Autodesk Inventor part; units mm, degrees
(part 3 of 6)
  line L1824 (13.0001, 24.773) -> (14.0001, 24.773)
  line L1825 (14.0001, 24.773) -> (14.0001, 25.773)
  line L1826 (14.0001, 25.773) -> (13.0001, 25.773)
  line L1827 (13.0001, 25.773) -> (13.0001, 24.773)
  line L1828 (13.8383, 24.773) -> (14.8383, 24.773)
  line L1829 (14.8383, 24.773) -> (14.8383, 25.773)
  line L1830 (14.8383, 25.773) -> (13.8383, 25.773)
  line L1831 (13.8383, 25.773) -> (13.8383, 24.773)
  line L1832 (14.6765, 24.773) -> (15.6765, 24.773)
  line L1833 (15.6765, 24.773) -> (15.6765, 25.773)
  line L1834 (15.6765, 25.773) -> (14.6765, 25.773)
  line L1835 (14.6765, 25.773) -> (14.6765, 24.773)
  line L1836 (15.4766, 24.773) -> (16.4766, 24.773)
  line L1837 (16.4766, 24.773) -> (16.4766, 25.773)
  line L1838 (16.4766, 25.773) -> (15.4766, 25.773)
  line L1839 (15.4766, 25.773) -> (15.4766, 24.773)
  line L1840 (15.9973, 24.773) -> (16.9973, 24.773)
  line L1841 (16.9973, 24.773) -> (16.9973, 25.773)
  line L1842 (16.9973, 25.773) -> (15.9973, 25.773)
  line L1843 (15.9973, 25.773) -> (15.9973, 24.773)
  line L1844 (17.153, 24.773) -> (18.153, 24.773)
  line L1845 (18.153, 24.773) -> (18.153, 25.773)
  line L1846 (18.153, 25.773) -> (17.153, 25.773)
  line L1847 (17.153, 25.773) -> (17.153, 24.773)
  line L1848 (17.915, 24.773) -> (18.915, 24.773)
  line L1849 (18.915, 24.773) -> (18.915, 25.773)
  line L1850 (18.915, 25.773) -> (17.915, 25.773)
  line L1851 (17.915, 25.773) -> (17.915, 24.773)
  line L1852 (18.677, 24.773) -> (19.677, 24.773)
  line L1853 (19.677, 24.773) -> (19.677, 25.773)
  line L1854 (19.677, 25.773) -> (18.677, 25.773)
  line L1855 (18.677, 25.773) -> (18.677, 24.773)
  line L1856 (19.2358, 24.773) -> (20.2358, 24.773)
  line L1857 (20.2358, 24.773) -> (20.2358, 25.773)
  line L1858 (20.2358, 25.773) -> (19.2358, 25.773)
  line L1859 (19.2358, 25.773) -> (19.2358, 24.773)
  line L1860 (19.8327, 24.773) -> (20.8327, 24.773)
  line L1861 (20.8327, 24.773) -> (20.8327, 25.773)
  line L1862 (20.8327, 25.773) -> (19.8327, 25.773)
  line L1863 (19.8327, 25.773) -> (19.8327, 24.773)
  line L1864 (20.4677, 24.773) -> (21.4677, 24.773)
  line L1865 (21.4677, 24.773) -> (21.4677, 25.773)
  line L1866 (21.4677, 25.773) -> (20.4677, 25.773)
  line L1867 (20.4677, 25.773) -> (20.4677, 24.773)
  line L1868 (21.471, 24.773) -> (22.471, 24.773)
  line L1869 (22.471, 24.773) -> (22.471, 25.773)
  line L1870 (22.471, 25.773) -> (21.471, 25.773)
  line L1871 (21.471, 25.773) -> (21.471, 24.773)
  line L1872 (12.9874, 24.7984) -> (13.9874, 24.7984)
  line L1873 (13.9874, 24.7984) -> (13.9874, 25.7984)
  line L1874 (13.9874, 25.7984) -> (12.9874, 25.7984)
  line L1875 (12.9874, 25.7984) -> (12.9874, 24.7984)
  line L1876 (13.8256, 24.7984) -> (14.8256, 24.7984)
  line L1877 (14.8256, 24.7984) -> (14.8256, 25.7984)
  line L1878 (14.8256, 25.7984) -> (13.8256, 25.7984)
  line L1879 (13.8256, 25.7984) -> (13.8256, 24.7984)
  line L1880 (14.6765, 24.7984) -> (15.6765, 24.7984)
  line L1881 (15.6765, 24.7984) -> (15.6765, 25.7984)
  line L1882 (15.6765, 25.7984) -> (14.6765, 25.7984)
  line L1883 (14.6765, 25.7984) -> (14.6765, 24.7984)
  line L1884 (15.4766, 24.7984) -> (16.4766, 24.7984)
  line L1885 (16.4766, 24.7984) -> (16.4766, 25.7984)
  line L1886 (16.4766, 25.7984) -> (15.4766, 25.7984)
  line L1887 (15.4766, 25.7984) -> (15.4766, 24.7984)
  line L1888 (15.9846, 24.7984) -> (16.9846, 24.7984)
  line L1889 (16.9846, 24.7984) -> (16.9846, 25.7984)
  line L1890 (16.9846, 25.7984) -> (15.9846, 25.7984)
  line L1891 (15.9846, 25.7984) -> (15.9846, 24.7984)
  line L1892 (17.1276, 24.7984) -> (18.1276, 24.7984)
  line L1893 (18.1276, 24.7984) -> (18.1276, 25.7984)
  line L1894 (18.1276, 25.7984) -> (17.1276, 25.7984)
  line L1895 (17.1276, 25.7984) -> (17.1276, 24.7984)
  line L1896 (17.915, 24.7984) -> (18.915, 24.7984)
  line L1897 (18.915, 24.7984) -> (18.915, 25.7984)
  line L1898 (18.915, 25.7984) -> (17.915, 25.7984)
  line L1899 (17.915, 25.7984) -> (17.915, 24.7984)
  line L1900 (18.677, 24.7984) -> (19.677, 24.7984)
  line L1901 (19.677, 24.7984) -> (19.677, 25.7984)
  line L1902 (19.677, 25.7984) -> (18.677, 25.7984)
  line L1903 (18.677, 25.7984) -> (18.677, 24.7984)
  line L1904 (19.2358, 24.7984) -> (20.2358, 24.7984)
  line L1905 (20.2358, 24.7984) -> (20.2358, 25.7984)
  line L1906 (20.2358, 25.7984) -> (19.2358, 25.7984)
  line L1907 (19.2358, 25.7984) -> (19.2358, 24.7984)
  line L1908 (19.8454, 24.7984) -> (20.8454, 24.7984)
  line L1909 (20.8454, 24.7984) -> (20.8454, 25.7984)
  line L1910 (20.8454, 25.7984) -> (19.8454, 25.7984)
  line L1911 (19.8454, 25.7984) -> (19.8454, 24.7984)
  line L1912 (20.4677, 24.7984) -> (21.4677, 24.7984)
  line L1913 (21.4677, 24.7984) -> (21.4677, 25.7984)
  line L1914 (21.4677, 25.7984) -> (20.4677, 25.7984)
  line L1915 (20.4677, 25.7984) -> (20.4677, 24.7984)
  line L1916 (21.471, 24.7984) -> (22.471, 24.7984)
  line L1917 (22.471, 24.7984) -> (22.471, 25.7984)
  line L1918 (22.471, 25.7984) -> (21.471, 25.7984)
  line L1919 (21.471, 25.7984) -> (21.471, 24.7984)
  line L1920 (12.9874, 24.8238) -> (13.9874, 24.8238)
  line L1921 (13.9874, 24.8238) -> (13.9874, 25.8238)
  line L1922 (13.9874, 25.8238) -> (12.9874, 25.8238)
  line L1923 (12.9874, 25.8238) -> (12.9874, 24.8238)
  line L1924 (13.8002, 24.8238) -> (14.8002, 24.8238)
  line L1925 (14.8002, 24.8238) -> (14.8002, 25.8238)
  line L1926 (14.8002, 25.8238) -> (13.8002, 25.8238)
  line L1927 (13.8002, 25.8238) -> (13.8002, 24.8238)
  line L1928 (14.6638, 24.8238) -> (15.6638, 24.8238)
  line L1929 (15.6638, 24.8238) -> (15.6638, 25.8238)
  line L1930 (15.6638, 25.8238) -> (14.6638, 25.8238)
  line L1931 (14.6638, 25.8238) -> (14.6638, 24.8238)
  line L1932 (15.4766, 24.8238) -> (16.4766, 24.8238)
  line L1933 (16.4766, 24.8238) -> (16.4766, 25.8238)
  line L1934 (16.4766, 25.8238) -> (15.4766, 25.8238)
  line L1935 (15.4766, 25.8238) -> (15.4766, 24.8238)
  line L1936 (15.9846, 24.8238) -> (16.9846, 24.8238)
  line L1937 (16.9846, 24.8238) -> (16.9846, 25.8238)
  line L1938 (16.9846, 25.8238) -> (15.9846, 25.8238)
  line L1939 (15.9846, 25.8238) -> (15.9846, 24.8238)
  line L1940 (17.1022, 24.8238) -> (18.1022, 24.8238)
  line L1941 (18.1022, 24.8238) -> (18.1022, 25.8238)
  line L1942 (18.1022, 25.8238) -> (17.1022, 25.8238)
  line L1943 (17.1022, 25.8238) -> (17.1022, 24.8238)
  line L1944 (17.915, 24.8238) -> (18.915, 24.8238)
  line L1945 (18.915, 24.8238) -> (18.915, 25.8238)
  line L1946 (18.915, 25.8238) -> (17.915, 25.8238)
  line L1947 (17.915, 25.8238) -> (17.915, 24.8238)
  line L1948 (18.677, 24.8238) -> (19.677, 24.8238)
  line L1949 (19.677, 24.8238) -> (19.677, 25.8238)
  line L1950 (19.677, 25.8238) -> (18.677, 25.8238)
  line L1951 (18.677, 25.8238) -> (18.677, 24.8238)
  line L1952 (19.2358, 24.8238) -> (20.2358, 24.8238)
  line L1953 (20.2358, 24.8238) -> (20.2358, 25.8238)
  line L1954 (20.2358, 25.8238) -> (19.2358, 25.8238)
  line L1955 (19.2358, 25.8238) -> (19.2358, 24.8238)
  line L1956 (19.8454, 24.8238) -> (20.8454, 24.8238)
  line L1957 (20.8454, 24.8238) -> (20.8454, 25.8238)
  line L1958 (20.8454, 25.8238) -> (19.8454, 25.8238)
  line L1959 (19.8454, 25.8238) -> (19.8454, 24.8238)
  line L1960 (20.4804, 24.8238) -> (21.4804, 24.8238)
  line L1961 (21.4804, 24.8238) -> (21.4804, 25.8238)
  line L1962 (21.4804, 25.8238) -> (20.4804, 25.8238)
  line L1963 (20.4804, 25.8238) -> (20.4804, 24.8238)
  line L1964 (21.471, 24.8238) -> (22.471, 24.8238)
  line L1965 (22.471, 24.8238) -> (22.471, 25.8238)
  line L1966 (22.471, 25.8238) -> (21.471, 25.8238)
  line L1967 (21.471, 25.8238) -> (21.471, 24.8238)
  line L1968 (12.9747, 24.8492) -> (13.9747, 24.8492)
  line L1969 (13.9747, 24.8492) -> (13.9747, 25.8492)
  line L1970 (13.9747, 25.8492) -> (12.9747, 25.8492)
  line L1971 (12.9747, 25.8492) -> (12.9747, 24.8492)
  line L1972 (13.7748, 24.8492) -> (14.7748, 24.8492)
  line L1973 (14.7748, 24.8492) -> (14.7748, 25.8492)
  line L1974 (14.7748, 25.8492) -> (13.7748, 25.8492)
  line L1975 (13.7748, 25.8492) -> (13.7748, 24.8492)
  line L1976 (14.6384, 24.8492) -> (15.6384, 24.8492)
  line L1977 (15.6384, 24.8492) -> (15.6384, 25.8492)
  line L1978 (15.6384, 25.8492) -> (14.6384, 25.8492)
  line L1979 (14.6384, 25.8492) -> (14.6384, 24.8492)
  line L1980 (15.7941, 24.8492) -> (16.7941, 24.8492)
  line L1981 (16.7941, 24.8492) -> (16.7941, 25.8492)
  line L1982 (16.7941, 25.8492) -> (15.7941, 25.8492)
  line L1983 (15.7941, 25.8492) -> (15.7941, 24.8492)
  line L1984 (17.1022, 24.8492) -> (18.1022, 24.8492)
  line L1985 (18.1022, 24.8492) -> (18.1022, 25.8492)
  line L1986 (18.1022, 25.8492) -> (17.1022, 25.8492)
  line L1987 (17.1022, 25.8492) -> (17.1022, 24.8492)
  line L1988 (17.9277, 24.8492) -> (18.9277, 24.8492)
  line L1989 (18.9277, 24.8492) -> (18.9277, 25.8492)
  line L1990 (18.9277, 25.8492) -> (17.9277, 25.8492)
  line L1991 (17.9277, 25.8492) -> (17.9277, 24.8492)
  line L1992 (18.677, 24.8492) -> (19.677, 24.8492)
  line L1993 (19.677, 24.8492) -> (19.677, 25.8492)
  line L1994 (19.677, 25.8492) -> (18.677, 25.8492)
  line L1995 (18.677, 25.8492) -> (18.677, 24.8492)
  line L1996 (19.2358, 24.8492) -> (20.2358, 24.8492)
  line L1997 (20.2358, 24.8492) -> (20.2358, 25.8492)
  line L1998 (20.2358, 25.8492) -> (19.2358, 25.8492)
  line L1999 (19.2358, 25.8492) -> (19.2358, 24.8492)
  line L2000 (19.8454, 24.8492) -> (20.8454, 24.8492)
  line L2001 (20.8454, 24.8492) -> (20.8454, 25.8492)
  line L2002 (20.8454, 25.8492) -> (19.8454, 25.8492)
  line L2003 (19.8454, 25.8492) -> (19.8454, 24.8492)
  line L2004 (20.4804, 24.8492) -> (21.4804, 24.8492)
  line L2005 (21.4804, 24.8492) -> (21.4804, 25.8492)
  line L2006 (21.4804, 25.8492) -> (20.4804, 25.8492)
  line L2007 (20.4804, 25.8492) -> (20.4804, 24.8492)
  line L2008 (21.471, 24.8492) -> (22.471, 24.8492)
  line L2009 (22.471, 24.8492) -> (22.471, 25.8492)
  line L2010 (22.471, 25.8492) -> (21.471, 25.8492)
  line L2011 (21.471, 25.8492) -> (21.471, 24.8492)
  line L2012 (12.962, 24.8746) -> (13.962, 24.8746)
  line L2013 (13.962, 24.8746) -> (13.962, 25.8746)
  line L2014 (13.962, 25.8746) -> (12.962, 25.8746)
  line L2015 (12.962, 25.8746) -> (12.962, 24.8746)
  line L2016 (13.7494, 24.8746) -> (14.7494, 24.8746)
  line L2017 (14.7494, 24.8746) -> (14.7494, 25.8746)
  line L2018 (14.7494, 25.8746) -> (13.7494, 25.8746)
  line L2019 (13.7494, 25.8746) -> (13.7494, 24.8746)
  line L2020 (14.6257, 24.8746) -> (15.6257, 24.8746)
  line L2021 (15.6257, 24.8746) -> (15.6257, 25.8746)
  line L2022 (15.6257, 25.8746) -> (14.6257, 25.8746)
  line L2023 (14.6257, 25.8746) -> (14.6257, 24.8746)
  line L2024 (15.8068, 24.8746) -> (16.8068, 24.8746)
  line L2025 (16.8068, 24.8746) -> (16.8068, 25.8746)
  line L2026 (16.8068, 25.8746) -> (15.8068, 25.8746)
  line L2027 (15.8068, 25.8746) -> (15.8068, 24.8746)
  line L2028 (17.0895, 24.8746) -> (18.0895, 24.8746)
  line L2029 (18.0895, 24.8746) -> (18.0895, 25.8746)
  line L2030 (18.0895, 25.8746) -> (17.0895, 25.8746)
  line L2031 (17.0895, 25.8746) -> (17.0895, 24.8746)
  line L2032 (17.9404, 24.8746) -> (18.9404, 24.8746)
  line L2033 (18.9404, 24.8746) -> (18.9404, 25.8746)
  line L2034 (18.9404, 25.8746) -> (17.9404, 25.8746)
  line L2035 (17.9404, 25.8746) -> (17.9404, 24.8746)
  line L2036 (18.677, 24.8746) -> (19.677, 24.8746)
  line L2037 (19.677, 24.8746) -> (19.677, 25.8746)
  line L2038 (19.677, 25.8746) -> (18.677, 25.8746)
  line L2039 (18.677, 25.8746) -> (18.677, 24.8746)
  line L2040 (19.2358, 24.8746) -> (20.2358, 24.8746)
  line L2041 (20.2358, 24.8746) -> (20.2358, 25.8746)
  line L2042 (20.2358, 25.8746) -> (19.2358, 25.8746)
  line L2043 (19.2358, 25.8746) -> (19.2358, 24.8746)
  line L2044 (19.8581, 24.8746) -> (20.8581, 24.8746)
  line L2045 (20.8581, 24.8746) -> (20.8581, 25.8746)
  line L2046 (20.8581, 25.8746) -> (19.8581, 25.8746)
  line L2047 (19.8581, 25.8746) -> (19.8581, 24.8746)
  line L2048 (20.4804, 24.8746) -> (21.4804, 24.8746)
  line L2049 (21.4804, 24.8746) -> (21.4804, 25.8746)
  line L2050 (21.4804, 25.8746) -> (20.4804, 25.8746)
  line L2051 (20.4804, 25.8746) -> (20.4804, 24.8746)
  line L2052 (21.4837, 24.8746) -> (22.4837, 24.8746)
  line L2053 (22.4837, 24.8746) -> (22.4837, 25.8746)
  line L2054 (22.4837, 25.8746) -> (21.4837, 25.8746)
  line L2055 (21.4837, 25.8746) -> (21.4837, 24.8746)
  line L2056 (12.9493, 24.9) -> (13.9493, 24.9)
  line L2057 (13.9493, 24.9) -> (13.9493, 25.9)
  line L2058 (13.9493, 25.9) -> (12.9493, 25.9)
  line L2059 (12.9493, 25.9) -> (12.9493, 24.9)
  line L2060 (13.7367, 24.9) -> (14.7367, 24.9)
  line L2061 (14.7367, 24.9) -> (14.7367, 25.9)
  line L2062 (14.7367, 25.9) -> (13.7367, 25.9)
  line L2063 (13.7367, 25.9) -> (13.7367, 24.9)
  line L2064 (14.6257, 24.9) -> (15.6257, 24.9)
  line L2065 (15.6257, 24.9) -> (15.6257, 25.9)
  line L2066 (15.6257, 25.9) -> (14.6257, 25.9)
  line L2067 (14.6257, 25.9) -> (14.6257, 24.9)
  line L2068 (15.8195, 24.9) -> (16.8195, 24.9)
  line L2069 (16.8195, 24.9) -> (16.8195, 25.9)
  line L2070 (16.8195, 25.9) -> (15.8195, 25.9)
  line L2071 (15.8195, 25.9) -> (15.8195, 24.9)
  line L2072 (17.0768, 24.9) -> (18.0768, 24.9)
  line L2073 (18.0768, 24.9) -> (18.0768, 25.9)
  line L2074 (18.0768, 25.9) -> (17.0768, 25.9)
  line L2075 (17.0768, 25.9) -> (17.0768, 24.9)
  line L2076 (17.9404, 24.9) -> (18.9404, 24.9)
  line L2077 (18.9404, 24.9) -> (18.9404, 25.9)
  line L2078 (18.9404, 25.9) -> (17.9404, 25.9)
  line L2079 (17.9404, 25.9) -> (17.9404, 24.9)
  line L2080 (18.677, 24.9) -> (19.677, 24.9)
  line L2081 (19.677, 24.9) -> (19.677, 25.9)
  line L2082 (19.677, 25.9) -> (18.677, 25.9)
  line L2083 (18.677, 25.9) -> (18.677, 24.9)
  line L2084 (19.2358, 24.9) -> (20.2358, 24.9)
  line L2085 (20.2358, 24.9) -> (20.2358, 25.9)
  line L2086 (20.2358, 25.9) -> (19.2358, 25.9)
  line L2087 (19.2358, 25.9) -> (19.2358, 24.9)
  line L2088 (19.8454, 24.9) -> (20.8454, 24.9)
  line L2089 (20.8454, 24.9) -> (20.8454, 25.9)
  line L2090 (20.8454, 25.9) -> (19.8454, 25.9)
  line L2091 (19.8454, 25.9) -> (19.8454, 24.9)
  line L2092 (20.4804, 24.9) -> (21.4804, 24.9)
  line L2093 (21.4804, 24.9) -> (21.4804, 25.9)
  line L2094 (21.4804, 25.9) -> (20.4804, 25.9)
  line L2095 (20.4804, 25.9) -> (20.4804, 24.9)
  line L2096 (21.471, 24.9) -> (22.471, 24.9)
  line L2097 (22.471, 24.9) -> (22.471, 25.9)
  line L2098 (22.471, 25.9) -> (21.471, 25.9)
  line L2099 (21.471, 25.9) -> (21.471, 24.9)
  line L2100 (12.9493, 24.9254) -> (13.9493, 24.9254)
  line L2101 (13.9493, 24.9254) -> (13.9493, 25.9254)
  line L2102 (13.9493, 25.9254) -> (12.9493, 25.9254)
  line L2103 (12.9493, 25.9254) -> (12.9493, 24.9254)
  line L2104 (13.7113, 24.9254) -> (14.7113, 24.9254)
  line L2105 (14.7113, 24.9254) -> (14.7113, 25.9254)
  line L2106 (14.7113, 25.9254) -> (13.7113, 25.9254)
  line L2107 (13.7113, 25.9254) -> (13.7113, 24.9254)
  line L2108 (14.6003, 24.9254) -> (15.6003, 24.9254)
  line L2109 (15.6003, 24.9254) -> (15.6003, 25.9254)
  line L2110 (15.6003, 25.9254) -> (14.6003, 25.9254)
  line L2111 (14.6003, 25.9254) -> (14.6003, 24.9254)
  line L2112 (15.8322, 24.9254) -> (16.8322, 24.9254)
  line L2113 (16.8322, 24.9254) -> (16.8322, 25.9254)
  line L2114 (16.8322, 25.9254) -> (15.8322, 25.9254)
  line L2115 (15.8322, 25.9254) -> (15.8322, 24.9254)
  line L2116 (17.0641, 24.9254) -> (18.0641, 24.9254)
  line L2117 (18.0641, 24.9254) -> (18.0641, 25.9254)
  line L2118 (18.0641, 25.9254) -> (17.0641, 25.9254)
  line L2119 (17.0641, 25.9254) -> (17.0641, 24.9254)
  line L2120 (17.9404, 24.9254) -> (18.9404, 24.9254)
  line L2121 (18.9404, 24.9254) -> (18.9404, 25.9254)
  line L2122 (18.9404, 25.9254) -> (17.9404, 25.9254)
  line L2123 (17.9404, 25.9254) -> (17.9404, 24.9254)
  line L2124 (18.677, 24.9254) -> (19.677, 24.9254)
  line L2125 (19.677, 24.9254) -> (19.677, 25.9254)
  line L2126 (19.677, 25.9254) -> (18.677, 25.9254)
  line L2127 (18.677, 25.9254) -> (18.677, 24.9254)
  line L2128 (19.2358, 24.9254) -> (20.2358, 24.9254)
  line L2129 (20.2358, 24.9254) -> (20.2358, 25.9254)
  line L2130 (20.2358, 25.9254) -> (19.2358, 25.9254)
  line L2131 (19.2358, 25.9254) -> (19.2358, 24.9254)
  line L2132 (19.8454, 24.9254) -> (20.8454, 24.9254)
  line L2133 (20.8454, 24.9254) -> (20.8454, 25.9254)
  line L2134 (20.8454, 25.9254) -> (19.8454, 25.9254)
  line L2135 (19.8454, 25.9254) -> (19.8454, 24.9254)
  line L2136 (20.4804, 24.9254) -> (21.4804, 24.9254)
  line L2137 (21.4804, 24.9254) -> (21.4804, 25.9254)
  line L2138 (21.4804, 25.9254) -> (20.4804, 25.9254)
  line L2139 (20.4804, 25.9254) -> (20.4804, 24.9254)
  line L2140 (21.4837, 24.9254) -> (22.4837, 24.9254)
  line L2141 (22.4837, 24.9254) -> (22.4837, 25.9254)
  line L2142 (22.4837, 25.9254) -> (21.4837, 25.9254)
  line L2143 (21.4837, 25.9254) -> (21.4837, 24.9254)
  line L2144 (12.9366, 24.9508) -> (13.9366, 24.9508)
  line L2145 (13.9366, 24.9508) -> (13.9366, 25.9508)
  line L2146 (13.9366, 25.9508) -> (12.9366, 25.9508)
  line L2147 (12.9366, 25.9508) -> (12.9366, 24.9508)
  line L2148 (13.6859, 24.9508) -> (14.6859, 24.9508)
  line L2149 (14.6859, 24.9508) -> (14.6859, 25.9508)
  line L2150 (14.6859, 25.9508) -> (13.6859, 25.9508)
  line L2151 (13.6859, 25.9508) -> (13.6859, 24.9508)
  line L2152 (14.5876, 24.9508) -> (15.5876, 24.9508)
  line L2153 (15.5876, 24.9508) -> (15.5876, 25.9508)
  line L2154 (15.5876, 25.9508) -> (14.5876, 25.9508)
  line L2155 (14.5876, 25.9508) -> (14.5876, 24.9508)
  line L2156 (15.8322, 24.9508) -> (16.8322, 24.9508)
  line L2157 (16.8322, 24.9508) -> (16.8322, 25.9508)
  line L2158 (16.8322, 25.9508) -> (15.8322, 25.9508)
  line L2159 (15.8322, 25.9508) -> (15.8322, 24.9508)
  line L2160 (17.0514, 24.9508) -> (18.0514, 24.9508)
  line L2161 (18.0514, 24.9508) -> (18.0514, 25.9508)
  line L2162 (18.0514, 25.9508) -> (17.0514, 25.9508)
  line L2163 (17.0514, 25.9508) -> (17.0514, 24.9508)
  line L2164 (17.9404, 24.9508) -> (18.9404, 24.9508)
  line L2165 (18.9404, 24.9508) -> (18.9404, 25.9508)
  line L2166 (18.9404, 25.9508) -> (17.9404, 25.9508)
  line L2167 (17.9404, 25.9508) -> (17.9404, 24.9508)
  line L2168 (18.677, 24.9508) -> (19.677, 24.9508)
  line L2169 (19.677, 24.9508) -> (19.677, 25.9508)
  line L2170 (19.677, 25.9508) -> (18.677, 25.9508)
  line L2171 (18.677, 25.9508) -> (18.677, 24.9508)
  line L2172 (19.2358, 24.9508) -> (20.2358, 24.9508)
  line L2173 (20.2358, 24.9508) -> (20.2358, 25.9508)
  line L2174 (20.2358, 25.9508) -> (19.2358, 25.9508)
  line L2175 (19.2358, 25.9508) -> (19.2358, 24.9508)
  line L2176 (19.8581, 24.9508) -> (20.8581, 24.9508)
  line L2177 (20.8581, 24.9508) -> (20.8581, 25.9508)
  line L2178 (20.8581, 25.9508) -> (19.8581, 25.9508)
  line L2179 (19.8581, 25.9508) -> (19.8581, 24.9508)
  line L2180 (20.4804, 24.9508) -> (21.4804, 24.9508)
  line L2181 (21.4804, 24.9508) -> (21.4804, 25.9508)
  line L2182 (21.4804, 25.9508) -> (20.4804, 25.9508)
  line L2183 (20.4804, 25.9508) -> (20.4804, 24.9508)
  line L2184 (21.4837, 24.9508) -> (22.4837, 24.9508)
  line L2185 (22.4837, 24.9508) -> (22.4837, 25.9508)
  line L2186 (22.4837, 25.9508) -> (21.4837, 25.9508)
  line L2187 (21.4837, 25.9508) -> (21.4837, 24.9508)
  line L2188 (12.9366, 24.9762) -> (13.9366, 24.9762)
  line L2189 (13.9366, 24.9762) -> (13.9366, 25.9762)
  line L2190 (13.9366, 25.9762) -> (12.9366, 25.9762)
  line L2191 (12.9366, 25.9762) -> (12.9366, 24.9762)
  line L2192 (13.6732, 24.9762) -> (14.6732, 24.9762)
  line L2193 (14.6732, 24.9762) -> (14.6732, 25.9762)
  line L2194 (14.6732, 25.9762) -> (13.6732, 25.9762)
  line L2195 (13.6732, 25.9762) -> (13.6732, 24.9762)
  line L2196 (14.5749, 24.9762) -> (15.5749, 24.9762)
  line L2197 (15.5749, 24.9762) -> (15.5749, 25.9762)
  line L2198 (15.5749, 25.9762) -> (14.5749, 25.9762)
  line L2199 (14.5749, 25.9762) -> (14.5749, 24.9762)
  line L2200 (15.8449, 24.9762) -> (16.8449, 24.9762)
  line L2201 (16.8449, 24.9762) -> (16.8449, 25.9762)
  line L2202 (16.8449, 25.9762) -> (15.8449, 25.9762)
  line L2203 (15.8449, 25.9762) -> (15.8449, 24.9762)
  line L2204 (17.0514, 24.9762) -> (18.0514, 24.9762)
  line L2205 (18.0514, 24.9762) -> (18.0514, 25.9762)
  line L2206 (18.0514, 25.9762) -> (17.0514, 25.9762)
  line L2207 (17.0514, 25.9762) -> (17.0514, 24.9762)
  line L2208 (17.9404, 24.9762) -> (18.9404, 24.9762)
  line L2209 (18.9404, 24.9762) -> (18.9404, 25.9762)
  line L2210 (18.9404, 25.9762) -> (17.9404, 25.9762)
  line L2211 (17.9404, 25.9762) -> (17.9404, 24.9762)
  line L2212 (18.677, 24.9762) -> (19.677, 24.9762)
  line L2213 (19.677, 24.9762) -> (19.677, 25.9762)
  line L2214 (19.677, 25.9762) -> (18.677, 25.9762)
  line L2215 (18.677, 25.9762) -> (18.677, 24.9762)
  line L2216 (19.2358, 24.9762) -> (20.2358, 24.9762)
  line L2217 (20.2358, 24.9762) -> (20.2358, 25.9762)
  line L2218 (20.2358, 25.9762) -> (19.2358, 25.9762)
  line L2219 (19.2358, 25.9762) -> (19.2358, 24.9762)
  line L2220 (19.8581, 24.9762) -> (20.8581, 24.9762)
  line L2221 (20.8581, 24.9762) -> (20.8581, 25.9762)
  line L2222 (20.8581, 25.9762) -> (19.8581, 25.9762)
  line L2223 (19.8581, 25.9762) -> (19.8581, 24.9762)
  line L2224 (20.4804, 24.9762) -> (21.4804, 24.9762)
  line L2225 (21.4804, 24.9762) -> (21.4804, 25.9762)
  line L2226 (21.4804, 25.9762) -> (20.4804, 25.9762)
  line L2227 (20.4804, 25.9762) -> (20.4804, 24.9762)
  line L2228 (21.4837, 24.9762) -> (22.4837, 24.9762)
  line L2229 (22.4837, 24.9762) -> (22.4837, 25.9762)
  line L2230 (22.4837, 25.9762) -> (21.4837, 25.9762)
  line L2231 (21.4837, 25.9762) -> (21.4837, 24.9762)
  line L2232 (12.9239, 25.0016) -> (13.9239, 25.0016)
  line L2233 (13.9239, 25.0016) -> (13.9239, 26.0016)
  line L2234 (13.9239, 26.0016) -> (12.9239, 26.0016)
  line L2235 (12.9239, 26.0016) -> (12.9239, 25.0016)
  line L2236 (13.6478, 25.0016) -> (14.6478, 25.0016)
  line L2237 (14.6478, 25.0016) -> (14.6478, 26.0016)
  line L2238 (14.6478, 26.0016) -> (13.6478, 26.0016)
  line L2239 (13.6478, 26.0016) -> (13.6478, 25.0016)
  line L2240 (14.5622, 25.0016) -> (15.5622, 25.0016)
  line L2241 (15.5622, 25.0016) -> (15.5622, 26.0016)
  line L2242 (15.5622, 26.0016) -> (14.5622, 26.0016)
  line L2243 (14.5622, 26.0016) -> (14.5622, 25.0016)
  line L2244 (15.8449, 25.0016) -> (16.8449, 25.0016)
  line L2245 (16.8449, 25.0016) -> (16.8449, 26.0016)
  line L2246 (16.8449, 26.0016) -> (15.8449, 26.0016)
  line L2247 (15.8449, 26.0016) -> (15.8449, 25.0016)
  line L2248 (16.8228, 25.0016) -> (17.8228, 25.0016)
  line L2249 (17.8228, 25.0016) -> (17.8228, 26.0016)
  line L2250 (17.8228, 26.0016) -> (16.8228, 26.0016)
  line L2251 (16.8228, 26.0016) -> (16.8228, 25.0016)
  line L2252 (17.4324, 25.0016) -> (18.4324, 25.0016)
  line L2253 (18.4324, 25.0016) -> (18.4324, 26.0016)
  line L2254 (18.4324, 26.0016) -> (17.4324, 26.0016)
  line L2255 (17.4324, 26.0016) -> (17.4324, 25.0016)
  line L2256 (17.9404, 25.0016) -> (18.9404, 25.0016)
  line L2257 (18.9404, 25.0016) -> (18.9404, 26.0016)
  line L2258 (18.9404, 26.0016) -> (17.9404, 26.0016)
  line L2259 (17.9404, 26.0016) -> (17.9404, 25.0016)
  line L2260 (18.677, 25.0016) -> (19.677, 25.0016)
  line L2261 (19.677, 25.0016) -> (19.677, 26.0016)
  line L2262 (19.677, 26.0016) -> (18.677, 26.0016)
  line L2263 (18.677, 26.0016) -> (18.677, 25.0016)
  line L2264 (19.2485, 25.0016) -> (20.2485, 25.0016)
  line L2265 (20.2485, 25.0016) -> (20.2485, 26.0016)
  line L2266 (20.2485, 26.0016) -> (19.2485, 26.0016)
  line L2267 (19.2485, 26.0016) -> (19.2485, 25.0016)
  line L2268 (19.8454, 25.0016) -> (20.8454, 25.0016)
  line L2269 (20.8454, 25.0016) -> (20.8454, 26.0016)
  line L2270 (20.8454, 26.0016) -> (19.8454, 26.0016)
  line L2271 (19.8454, 26.0016) -> (19.8454, 25.0016)
  line L2272 (20.4804, 25.0016) -> (21.4804, 25.0016)
  line L2273 (21.4804, 25.0016) -> (21.4804, 26.0016)
  line L2274 (21.4804, 26.0016) -> (20.4804, 26.0016)
  line L2275 (20.4804, 26.0016) -> (20.4804, 25.0016)
  line L2276 (21.4837, 25.0016) -> (22.4837, 25.0016)
  line L2277 (22.4837, 25.0016) -> (22.4837, 26.0016)
  line L2278 (22.4837, 26.0016) -> (21.4837, 26.0016)
  line L2279 (21.4837, 26.0016) -> (21.4837, 25.0016)
  line L2280 (12.9239, 25.027) -> (13.9239, 25.027)
  line L2281 (13.9239, 25.027) -> (13.9239, 26.027)
  line L2282 (13.9239, 26.027) -> (12.9239, 26.027)
  line L2283 (12.9239, 26.027) -> (12.9239, 25.027)
  line L2284 (13.6224, 25.027) -> (14.6224, 25.027)
  line L2285 (14.6224, 25.027) -> (14.6224, 26.027)
  line L2286 (14.6224, 26.027) -> (13.6224, 26.027)
  line L2287 (13.6224, 26.027) -> (13.6224, 25.027)
  line L2288 (14.5495, 25.027) -> (15.5495, 25.027)
  line L2289 (15.5495, 25.027) -> (15.5495, 26.027)
  line L2290 (15.5495, 26.027) -> (14.5495, 26.027)
  line L2291 (14.5495, 26.027) -> (14.5495, 25.027)
  line L2292 (15.5528, 25.027) -> (16.5528, 25.027)
  line L2293 (16.5528, 25.027) -> (16.5528, 26.027)
  line L2294 (16.5528, 26.027) -> (15.5528, 26.027)
  line L2295 (15.5528, 26.027) -> (15.5528, 25.027)
  line L2296 (16.1751, 25.027) -> (17.1751, 25.027)
  line L2297 (17.1751, 25.027) -> (17.1751, 26.027)
  line L2298 (17.1751, 26.027) -> (16.1751, 26.027)
  line L2299 (16.1751, 26.027) -> (16.1751, 25.027)
  line L2300 (16.7974, 25.027) -> (17.7974, 25.027)
  line L2301 (17.7974, 25.027) -> (17.7974, 26.027)
  line L2302 (17.7974, 26.027) -> (16.7974, 26.027)
  line L2303 (16.7974, 26.027) -> (16.7974, 25.027)
  line L2304 (17.4832, 25.027) -> (18.4832, 25.027)
  line L2305 (18.4832, 25.027) -> (18.4832, 26.027)
  line L2306 (18.4832, 26.027) -> (17.4832, 26.027)
  line L2307 (17.4832, 26.027) -> (17.4832, 25.027)
  line L2308 (17.9404, 25.027) -> (18.9404, 25.027)
  line L2309 (18.9404, 25.027) -> (18.9404, 26.027)
  line L2310 (18.9404, 26.027) -> (17.9404, 26.027)
  line L2311 (17.9404, 26.027) -> (17.9404, 25.027)
  line L2312 (18.677, 25.027) -> (19.677, 25.027)
  line L2313 (19.677, 25.027) -> (19.677, 26.027)
  line L2314 (19.677, 26.027) -> (18.677, 26.027)
  line L2315 (18.677, 26.027) -> (18.677, 25.027)
  line L2316 (19.2485, 25.027) -> (20.2485, 25.027)
  line L2317 (20.2485, 25.027) -> (20.2485, 26.027)
  line L2318 (20.2485, 26.027) -> (19.2485, 26.027)
  line L2319 (19.2485, 26.027) -> (19.2485, 25.027)
  line L2320 (19.8581, 25.027) -> (20.8581, 25.027)
  line L2321 (20.8581, 25.027) -> (20.8581, 26.027)
  line L2322 (20.8581, 26.027) -> (19.8581, 26.027)
  line L2323 (19.8581, 26.027) -> (19.8581, 25.027)
  line L2324 (20.4804, 25.027) -> (21.4804, 25.027)
  line L2325 (21.4804, 25.027) -> (21.4804, 26.027)
  line L2326 (21.4804, 26.027) -> (20.4804, 26.027)
  line L2327 (20.4804, 26.027) -> (20.4804, 25.027)
  line L2328 (21.4964, 25.027) -> (22.4964, 25.027)
  line L2329 (22.4964, 25.027) -> (22.4964, 26.027)
  line L2330 (22.4964, 26.027) -> (21.4964, 26.027)
  line L2331 (21.4964, 26.027) -> (21.4964, 25.027)
  line L2332 (12.9112, 25.0524) -> (13.9112, 25.0524)
  line L2333 (13.9112, 25.0524) -> (13.9112, 26.0524)
  line L2334 (13.9112, 26.0524) -> (12.9112, 26.0524)
  line L2335 (12.9112, 26.0524) -> (12.9112, 25.0524)
  line L2336 (13.597, 25.0524) -> (14.597, 25.0524)
  line L2337 (14.597, 25.0524) -> (14.597, 26.0524)
  line L2338 (14.597, 26.0524) -> (13.597, 26.0524)
  line L2339 (13.597, 26.0524) -> (13.597, 25.0524)
  line L2340 (14.5241, 25.0524) -> (15.5241, 25.0524)
  line L2341 (15.5241, 25.0524) -> (15.5241, 26.0524)
  line L2342 (15.5241, 26.0524) -> (14.5241, 26.0524)
  line L2343 (14.5241, 26.0524) -> (14.5241, 25.0524)
  line L2344 (15.5274, 25.0524) -> (16.5274, 25.0524)
  line L2345 (16.5274, 25.0524) -> (16.5274, 26.0524)
  line L2346 (16.5274, 26.0524) -> (15.5274, 26.0524)
  line L2347 (15.5274, 26.0524) -> (15.5274, 25.0524)
  line L2348 (16.2005, 25.0524) -> (17.2005, 25.0524)
  line L2349 (17.2005, 25.0524) -> (17.2005, 26.0524)
  line L2350 (17.2005, 26.0524) -> (16.2005, 26.0524)
  line L2351 (16.2005, 26.0524) -> (16.2005, 25.0524)
  line L2352 (16.772, 25.0524) -> (17.772, 25.0524)
  line L2353 (17.772, 25.0524) -> (17.772, 26.0524)
  line L2354 (17.772, 26.0524) -> (16.772, 26.0524)
  line L2355 (16.772, 26.0524) -> (16.772, 25.0524)
  line L2356 (17.9404, 25.0524) -> (18.9404, 25.0524)
  line L2357 (18.9404, 25.0524) -> (18.9404, 26.0524)
  line L2358 (18.9404, 26.0524) -> (17.9404, 26.0524)
  line L2359 (17.9404, 26.0524) -> (17.9404, 25.0524)
  line L2360 (18.677, 25.0524) -> (19.677, 25.0524)
  line L2361 (19.677, 25.0524) -> (19.677, 26.0524)
  line L2362 (19.677, 26.0524) -> (18.677, 26.0524)
  line L2363 (18.677, 26.0524) -> (18.677, 25.0524)
  line L2364 (19.2485, 25.0524) -> (20.2485, 25.0524)
  line L2365 (20.2485, 25.0524) -> (20.2485, 26.0524)
  line L2366 (20.2485, 26.0524) -> (19.2485, 26.0524)
  line L2367 (19.2485, 26.0524) -> (19.2485, 25.0524)
  line L2368 (19.8581, 25.0524) -> (20.8581, 25.0524)
  line L2369 (20.8581, 25.0524) -> (20.8581, 26.0524)
  line L2370 (20.8581, 26.0524) -> (19.8581, 26.0524)
  line L2371 (19.8581, 26.0524) -> (19.8581, 25.0524)
  line L2372 (20.4804, 25.0524) -> (21.4804, 25.0524)
  line L2373 (21.4804, 25.0524) -> (21.4804, 26.0524)
  line L2374 (21.4804, 26.0524) -> (20.4804, 26.0524)
  line L2375 (20.4804, 26.0524) -> (20.4804, 25.0524)
  line L2376 (21.4837, 25.0524) -> (22.4837, 25.0524)
  line L2377 (22.4837, 25.0524) -> (22.4837, 26.0524)
  line L2378 (22.4837, 26.0524) -> (21.4837, 26.0524)
  line L2379 (21.4837, 26.0524) -> (21.4837, 25.0524)
  line L2380 (12.9112, 25.0778) -> (13.9112, 25.0778)
  line L2381 (13.9112, 25.0778) -> (13.9112, 26.0778)
  line L2382 (13.9112, 26.0778) -> (12.9112, 26.0778)
  line L2383 (12.9112, 26.0778) -> (12.9112, 25.0778)
  line L2384 (13.5843, 25.0778) -> (14.5843, 25.0778)
  line L2385 (14.5843, 25.0778) -> (14.5843, 26.0778)
  line L2386 (14.5843, 26.0778) -> (13.5843, 26.0778)
  line L2387 (13.5843, 26.0778) -> (13.5843, 25.0778)
  line L2388 (14.5241, 25.0778) -> (15.5241, 25.0778)
  line L2389 (15.5241, 25.0778) -> (15.5241, 26.0778)
  line L2390 (15.5241, 26.0778) -> (14.5241, 26.0778)
  line L2391 (14.5241, 26.0778) -> (14.5241, 25.0778)
  line L2392 (15.5147, 25.0778) -> (16.5147, 25.0778)
  line L2393 (16.5147, 25.0778) -> (16.5147, 26.0778)
  line L2394 (16.5147, 26.0778) -> (15.5147, 26.0778)
  line L2395 (15.5147, 26.0778) -> (15.5147, 25.0778)
  line L2396 (16.2005, 25.0778) -> (17.2005, 25.0778)
  line L2397 (17.2005, 25.0778) -> (17.2005, 26.0778)
  line L2398 (17.2005, 26.0778) -> (16.2005, 26.0778)
  line L2399 (16.2005, 26.0778) -> (16.2005, 25.0778)
  line L2400 (16.7466, 25.0778) -> (17.7466, 25.0778)
  line L2401 (17.7466, 25.0778) -> (17.7466, 26.0778)
  line L2402 (17.7466, 26.0778) -> (16.7466, 26.0778)
  line L2403 (16.7466, 26.0778) -> (16.7466, 25.0778)
  line L2404 (17.9404, 25.0778) -> (18.9404, 25.0778)
  line L2405 (18.9404, 25.0778) -> (18.9404, 26.0778)
  line L2406 (18.9404, 26.0778) -> (17.9404, 26.0778)
  line L2407 (17.9404, 26.0778) -> (17.9404, 25.0778)
  line L2408 (18.677, 25.0778) -> (19.677, 25.0778)
  line L2409 (19.677, 25.0778) -> (19.677, 26.0778)
  line L2410 (19.677, 26.0778) -> (18.677, 26.0778)
  line L2411 (18.677, 26.0778) -> (18.677, 25.0778)
  line L2412 (19.2485, 25.0778) -> (20.2485, 25.0778)
  line L2413 (20.2485, 25.0778) -> (20.2485, 26.0778)
  line L2414 (20.2485, 26.0778) -> (19.2485, 26.0778)
  line L2415 (19.2485, 26.0778) -> (19.2485, 25.0778)
  line L2416 (19.8581, 25.0778) -> (20.8581, 25.0778)
  line L2417 (20.8581, 25.0778) -> (20.8581, 26.0778)
  line L2418 (20.8581, 26.0778) -> (19.8581, 26.0778)
  line L2419 (19.8581, 26.0778) -> (19.8581, 25.0778)
  line L2420 (20.4804, 25.0778) -> (21.4804, 25.0778)
  line L2421 (21.4804, 25.0778) -> (21.4804, 26.0778)
  line L2422 (21.4804, 26.0778) -> (20.4804, 26.0778)
  line L2423 (20.4804, 26.0778) -> (20.4804, 25.0778)
  line L2424 (21.4964, 25.0778) -> (22.4964, 25.0778)
  line L2425 (22.4964, 25.0778) -> (22.4964, 26.0778)
  line L2426 (22.4964, 26.0778) -> (21.4964, 26.0778)
  line L2427 (21.4964, 26.0778) -> (21.4964, 25.0778)
  line L2428 (12.8985, 25.1032) -> (13.8985, 25.1032)
  line L2429 (13.8985, 25.1032) -> (13.8985, 26.1032)
  line L2430 (13.8985, 26.1032) -> (12.8985, 26.1032)
  line L2431 (12.8985, 26.1032) -> (12.8985, 25.1032)
  line L2432 (13.5589, 25.1032) -> (14.5589, 25.1032)
  line L2433 (14.5589, 25.1032) -> (14.5589, 26.1032)
  line L2434 (14.5589, 26.1032) -> (13.5589, 26.1032)
  line L2435 (13.5589, 26.1032) -> (13.5589, 25.1032)
  line L2436 (14.4987, 25.1032) -> (15.4987, 25.1032)
  line L2437 (15.4987, 25.1032) -> (15.4987, 26.1032)
  line L2438 (15.4987, 26.1032) -> (14.4987, 26.1032)
  line L2439 (14.4987, 26.1032) -> (14.4987, 25.1032)
  line L2440 (15.5147, 25.1032) -> (16.5147, 25.1032)
  line L2441 (16.5147, 25.1032) -> (16.5147, 26.1032)
  line L2442 (16.5147, 26.1032) -> (15.5147, 26.1032)
  line L2443 (15.5147, 26.1032) -> (15.5147, 25.1032)
  line L2444 (16.2132, 25.1032) -> (17.2132, 25.1032)
  line L2445 (17.2132, 25.1032) -> (17.2132, 26.1032)
  line L2446 (17.2132, 26.1032) -> (16.2132, 26.1032)
  line L2447 (16.2132, 26.1032) -> (16.2132, 25.1032)
  line L2448 (16.7466, 25.1032) -> (17.7466, 25.1032)
  line L2449 (17.7466, 25.1032) -> (17.7466, 26.1032)
  line L2450 (17.7466, 26.1032) -> (16.7466, 26.1032)
  line L2451 (16.7466, 26.1032) -> (16.7466, 25.1032)
  line L2452 (17.9404, 25.1032) -> (18.9404, 25.1032)
  line L2453 (18.9404, 25.1032) -> (18.9404, 26.1032)
  line L2454 (18.9404, 26.1032) -> (17.9404, 26.1032)
  line L2455 (17.9404, 26.1032) -> (17.9404, 25.1032)
  line L2456 (18.677, 25.1032) -> (19.677, 25.1032)
  line L2457 (19.677, 25.1032) -> (19.677, 26.1032)
  line L2458 (19.677, 26.1032) -> (18.677, 26.1032)
  line L2459 (18.677, 26.1032) -> (18.677, 25.1032)
  line L2460 (19.2485, 25.1032) -> (20.2485, 25.1032)
  line L2461 (20.2485, 25.1032) -> (20.2485, 26.1032)
  line L2462 (20.2485, 26.1032) -> (19.2485, 26.1032)
  line L2463 (19.2485, 26.1032) -> (19.2485, 25.1032)
  line L2464 (19.8581, 25.1032) -> (20.8581, 25.1032)
  line L2465 (20.8581, 25.1032) -> (20.8581, 26.1032)
  line L2466 (20.8581, 26.1032) -> (19.8581, 26.1032)
  line L2467 (19.8581, 26.1032) -> (19.8581, 25.1032)
  line L2468 (20.4804, 25.1032) -> (21.4804, 25.1032)
  line L2469 (21.4804, 25.1032) -> (21.4804, 26.1032)
  line L2470 (21.4804, 26.1032) -> (20.4804, 26.1032)
  line L2471 (20.4804, 26.1032) -> (20.4804, 25.1032)
  line L2472 (21.3059, 25.1032) -> (22.3059, 25.1032)
  line L2473 (22.3059, 25.1032) -> (22.3059, 26.1032)
  line L2474 (22.3059, 26.1032) -> (21.3059, 26.1032)
  line L2475 (21.3059, 26.1032) -> (21.3059, 25.1032)
  line L2476 (21.6869, 25.1032) -> (22.6869, 25.1032)
  line L2477 (22.6869, 25.1032) -> (22.6869, 26.1032)
  line L2478 (22.6869, 26.1032) -> (21.6869, 26.1032)
  line L2479 (21.6869, 26.1032) -> (21.6869, 25.1032)
  line L2480 (12.8985, 25.1286) -> (13.8985, 25.1286)
  line L2481 (13.8985, 25.1286) -> (13.8985, 26.1286)
  line L2482 (13.8985, 26.1286) -> (12.8985, 26.1286)
  line L2483 (12.8985, 26.1286) -> (12.8985, 25.1286)
  line L2484 (13.5335, 25.1286) -> (14.5335, 25.1286)
  line L2485 (14.5335, 25.1286) -> (14.5335, 26.1286)
  line L2486 (14.5335, 26.1286) -> (13.5335, 26.1286)
  line L2487 (13.5335, 26.1286) -> (13.5335, 25.1286)
  line L2488 (14.486, 25.1286) -> (15.486, 25.1286)
  line L2489 (15.486, 25.1286) -> (15.486, 26.1286)
  line L2490 (15.486, 26.1286) -> (14.486, 26.1286)
  line L2491 (14.486, 26.1286) -> (14.486, 25.1286)
  line L2492 (15.502, 25.1286) -> (16.502, 25.1286)
  line L2493 (16.502, 25.1286) -> (16.502, 26.1286)
  line L2494 (16.502, 26.1286) -> (15.502, 26.1286)
  line L2495 (15.502, 26.1286) -> (15.502, 25.1286)
  line L2496 (16.2386, 25.1286) -> (17.2386, 25.1286)
  line L2497 (17.2386, 25.1286) -> (17.2386, 26.1286)
  line L2498 (17.2386, 26.1286) -> (16.2386, 26.1286)
  line L2499 (16.2386, 26.1286) -> (16.2386, 25.1286)
  line L2500 (16.7466, 25.1286) -> (17.7466, 25.1286)
  line L2501 (17.7466, 25.1286) -> (17.7466, 26.1286)
  line L2502 (17.7466, 26.1286) -> (16.7466, 26.1286)
  line L2503 (16.7466, 26.1286) -> (16.7466, 25.1286)
  line L2504 (17.9404, 25.1286) -> (18.9404, 25.1286)
  line L2505 (18.9404, 25.1286) -> (18.9404, 26.1286)
  line L2506 (18.9404, 26.1286) -> (17.9404, 26.1286)
  line L2507 (17.9404, 26.1286) -> (17.9404, 25.1286)
  line L2508 (18.677, 25.1286) -> (19.677, 25.1286)
  line L2509 (19.677, 25.1286) -> (19.677, 26.1286)
  line L2510 (19.677, 26.1286) -> (18.677, 26.1286)
  line L2511 (18.677, 26.1286) -> (18.677, 25.1286)
  line L2512 (19.2485, 25.1286) -> (20.2485, 25.1286)
  line L2513 (20.2485, 25.1286) -> (20.2485, 26.1286)
  line L2514 (20.2485, 26.1286) -> (19.2485, 26.1286)
  line L2515 (19.2485, 26.1286) -> (19.2485, 25.1286)
  line L2516 (19.8581, 25.1286) -> (20.8581, 25.1286)
  line L2517 (20.8581, 25.1286) -> (20.8581, 26.1286)
  line L2518 (20.8581, 26.1286) -> (19.8581, 26.1286)
  line L2519 (19.8581, 26.1286) -> (19.8581, 25.1286)
  line L2520 (20.4804, 25.1286) -> (21.4804, 25.1286)
  line L2521 (21.4804, 25.1286) -> (21.4804, 26.1286)
  line L2522 (21.4804, 26.1286) -> (20.4804, 26.1286)
  line L2523 (20.4804, 26.1286) -> (20.4804, 25.1286)
  line L2524 (21.2932, 25.1286) -> (22.2932, 25.1286)
  line L2525 (22.2932, 25.1286) -> (22.2932, 26.1286)
  line L2526 (22.2932, 26.1286) -> (21.2932, 26.1286)
  line L2527 (21.2932, 26.1286) -> (21.2932, 25.1286)
  line L2528 (21.6996, 25.1286) -> (22.6996, 25.1286)
  line L2529 (22.6996, 25.1286) -> (22.6996, 26.1286)
  line L2530 (22.6996, 26.1286) -> (21.6996, 26.1286)
  line L2531 (21.6996, 26.1286) -> (21.6996, 25.1286)
  line L2532 (12.8858, 25.154) -> (13.8858, 25.154)
  line L2533 (13.8858, 25.154) -> (13.8858, 26.154)
  line L2534 (13.8858, 26.154) -> (12.8858, 26.154)
  line L2535 (12.8858, 26.154) -> (12.8858, 25.154)
  line L2536 (13.5208, 25.154) -> (14.5208, 25.154)
  line L2537 (14.5208, 25.154) -> (14.5208, 26.154)
  line L2538 (14.5208, 26.154) -> (13.5208, 26.154)
  line L2539 (13.5208, 26.154) -> (13.5208, 25.154)
  line L2540 (14.4606, 25.154) -> (15.4606, 25.154)
  line L2541 (15.4606, 25.154) -> (15.4606, 26.154)
  line L2542 (15.4606, 26.154) -> (14.4606, 26.154)
  line L2543 (14.4606, 26.154) -> (14.4606, 25.154)
  line L2544 (15.502, 25.154) -> (16.502, 25.154)
  line L2545 (16.502, 25.154) -> (16.502, 26.154)
  line L2546 (16.502, 26.154) -> (15.502, 26.154)
  line L2547 (15.502, 26.154) -> (15.502, 25.154)
  line L2548 (16.2386, 25.154) -> (17.2386, 25.154)
  line L2549 (17.2386, 25.154) -> (17.2386, 26.154)
  line L2550 (17.2386, 26.154) -> (16.2386, 26.154)
  line L2551 (16.2386, 26.154) -> (16.2386, 25.154)
  line L2552 (16.7339, 25.154) -> (17.7339, 25.154)
  line L2553 (17.7339, 25.154) -> (17.7339, 26.154)
  line L2554 (17.7339, 26.154) -> (16.7339, 26.154)
  line L2555 (16.7339, 26.154) -> (16.7339, 25.154)
  line L2556 (17.9531, 25.154) -> (18.9531, 25.154)
  line L2557 (18.9531, 25.154) -> (18.9531, 26.154)
  line L2558 (18.9531, 26.154) -> (17.9531, 26.154)
  line L2559 (17.9531, 26.154) -> (17.9531, 25.154)
  line L2560 (18.677, 25.154) -> (19.677, 25.154)
  line L2561 (19.677, 25.154) -> (19.677, 26.154)
  line L2562 (19.677, 26.154) -> (18.677, 26.154)
  line L2563 (18.677, 26.154) -> (18.677, 25.154)
  line L2564 (19.2485, 25.154) -> (20.2485, 25.154)
  line L2565 (20.2485, 25.154) -> (20.2485, 26.154)
  line L2566 (20.2485, 26.154) -> (19.2485, 26.154)
  line L2567 (19.2485, 26.154) -> (19.2485, 25.154)
  line L2568 (19.8581, 25.154) -> (20.8581, 25.154)
  line L2569 (20.8581, 25.154) -> (20.8581, 26.154)
  line L2570 (20.8581, 26.154) -> (19.8581, 26.154)
  line L2571 (19.8581, 26.154) -> (19.8581, 25.154)
  line L2572 (20.4804, 25.154) -> (21.4804, 25.154)
  line L2573 (21.4804, 25.154) -> (21.4804, 26.154)
  line L2574 (21.4804, 26.154) -> (20.4804, 26.154)
  line L2575 (20.4804, 26.154) -> (20.4804, 25.154)
  line L2576 (21.2932, 25.154) -> (22.2932, 25.154)
  line L2577 (22.2932, 25.154) -> (22.2932, 26.154)
  line L2578 (22.2932, 26.154) -> (21.2932, 26.154)
  line L2579 (21.2932, 26.154) -> (21.2932, 25.154)
  line L2580 (21.7123, 25.154) -> (22.7123, 25.154)
  line L2581 (22.7123, 25.154) -> (22.7123, 26.154)
  line L2582 (22.7123, 26.154) -> (21.7123, 26.154)
  line L2583 (21.7123, 26.154) -> (21.7123, 25.154)
  line L2584 (12.8858, 25.1794) -> (13.8858, 25.1794)
  line L2585 (13.8858, 25.1794) -> (13.8858, 26.1794)
  line L2586 (13.8858, 26.1794) -> (12.8858, 26.1794)
  line L2587 (12.8858, 26.1794) -> (12.8858, 25.1794)
  line L2588 (13.4954, 25.1794) -> (14.4954, 25.1794)
  line L2589 (14.4954, 25.1794) -> (14.4954, 26.1794)
  line L2590 (14.4954, 26.1794) -> (13.4954, 26.1794)
  line L2591 (13.4954, 26.1794) -> (13.4954, 25.1794)
  line L2592 (14.4733, 25.1794) -> (15.4733, 25.1794)
  line L2593 (15.4733, 25.1794) -> (15.4733, 26.1794)
  line L2594 (15.4733, 26.1794) -> (14.4733, 26.1794)
  line L2595 (14.4733, 26.1794) -> (14.4733, 25.1794)
  line L2596 (15.502, 25.1794) -> (16.502, 25.1794)
  line L2597 (16.502, 25.1794) -> (16.502, 26.1794)
  line L2598 (16.502, 26.1794) -> (15.502, 26.1794)
  line L2599 (15.502, 26.1794) -> (15.502, 25.1794)
  line L2600 (16.2386, 25.1794) -> (17.2386, 25.1794)
  line L2601 (17.2386, 25.1794) -> (17.2386, 26.1794)
  line L2602 (17.2386, 26.1794) -> (16.2386, 26.1794)
  line L2603 (16.2386, 26.1794) -> (16.2386, 25.1794)
  line L2604 (16.7339, 25.1794) -> (17.7339, 25.1794)
  line L2605 (17.7339, 25.1794) -> (17.7339, 26.1794)
  line L2606 (17.7339, 26.1794) -> (16.7339, 26.1794)
  line L2607 (16.7339, 26.1794) -> (16.7339, 25.1794)
  line L2608 (17.9531, 25.1794) -> (18.9531, 25.1794)
  line L2609 (18.9531, 25.1794) -> (18.9531, 26.1794)
  line L2610 (18.9531, 26.1794) -> (17.9531, 26.1794)
  line L2611 (17.9531, 26.1794) -> (17.9531, 25.1794)
  line L2612 (18.677, 25.1794) -> (19.677, 25.1794)
  line L2613 (19.677, 25.1794) -> (19.677, 26.1794)
  line L2614 (19.677, 26.1794) -> (18.677, 26.1794)
  line L2615 (18.677, 26.1794) -> (18.677, 25.1794)
  line L2616 (19.2485, 25.1794) -> (20.2485, 25.1794)
  line L2617 (20.2485, 25.1794) -> (20.2485, 26.1794)
  line L2618 (20.2485, 26.1794) -> (19.2485, 26.1794)
  line L2619 (19.2485, 26.1794) -> (19.2485, 25.1794)
  line L2620 (19.8708, 25.1794) -> (20.8708, 25.1794)
  line L2621 (20.8708, 25.1794) -> (20.8708, 26.1794)
  line L2622 (20.8708, 26.1794) -> (19.8708, 26.1794)
  line L2623 (19.8708, 26.1794) -> (19.8708, 25.1794)
  line L2624 (20.4804, 25.1794) -> (21.4804, 25.1794)
  line L2625 (21.4804, 25.1794) -> (21.4804, 26.1794)
  line L2626 (21.4804, 26.1794) -> (20.4804, 26.1794)
  line L2627 (20.4804, 26.1794) -> (20.4804, 25.1794)
  line L2628 (21.2805, 25.1794) -> (22.2805, 25.1794)
  line L2629 (22.2805, 25.1794) -> (22.2805, 26.1794)
  line L2630 (22.2805, 26.1794) -> (21.2805, 26.1794)
  line L2631 (21.2805, 26.1794) -> (21.2805, 25.1794)
  line L2632 (21.725, 25.1794) -> (22.725, 25.1794)
  line L2633 (22.725, 25.1794) -> (22.725, 26.1794)
  line L2634 (22.725, 26.1794) -> (21.725, 26.1794)
  line L2635 (21.725, 26.1794) -> (21.725, 25.1794)
  line L2636 (12.8731, 25.2048) -> (13.8731, 25.2048)
  line L2637 (13.8731, 25.2048) -> (13.8731, 26.2048)
  line L2638 (13.8731, 26.2048) -> (12.8731, 26.2048)
  line L2639 (12.8731, 26.2048) -> (12.8731, 25.2048)
  line L2640 (13.47, 25.2048) -> (14.47, 25.2048)
  line L2641 (14.47, 25.2048) -> (14.47, 26.2048)
  line L2642 (14.47, 26.2048) -> (13.47, 26.2048)
  line L2643 (13.47, 26.2048) -> (13.47, 25.2048)
  line L2644 (14.4987, 25.2048) -> (15.4987, 25.2048)
  line L2645 (15.4987, 25.2048) -> (15.4987, 26.2048)
  line L2646 (15.4987, 26.2048) -> (14.4987, 26.2048)
  line L2647 (14.4987, 26.2048) -> (14.4987, 25.2048)
  line L2648 (15.502, 25.2048) -> (16.502, 25.2048)
  line L2649 (16.502, 25.2048) -> (16.502, 26.2048)
  line L2650 (16.502, 26.2048) -> (15.502, 26.2048)
  line L2651 (15.502, 26.2048) -> (15.502, 25.2048)
  line L2652 (16.2386, 25.2048) -> (17.2386, 25.2048)
  line L2653 (17.2386, 25.2048) -> (17.2386, 26.2048)
  line L2654 (17.2386, 26.2048) -> (16.2386, 26.2048)
  line L2655 (16.2386, 26.2048) -> (16.2386, 25.2048)
  line L2656 (16.7339, 25.2048) -> (17.7339, 25.2048)
  line L2657 (17.7339, 25.2048) -> (17.7339, 26.2048)
  line L2658 (17.7339, 26.2048) -> (16.7339, 26.2048)
  line L2659 (16.7339, 26.2048) -> (16.7339, 25.2048)
  line L2660 (17.9531, 25.2048) -> (18.9531, 25.2048)
  line L2661 (18.9531, 25.2048) -> (18.9531, 26.2048)
  line L2662 (18.9531, 26.2048) -> (17.9531, 26.2048)
  line L2663 (17.9531, 26.2048) -> (17.9531, 25.2048)
  line L2664 (18.677, 25.2048) -> (19.677, 25.2048)
  line L2665 (19.677, 25.2048) -> (19.677, 26.2048)
  line L2666 (19.677, 26.2048) -> (18.677, 26.2048)
  line L2667 (18.677, 26.2048) -> (18.677, 25.2048)
  line L2668 (19.2612, 25.2048) -> (20.2612, 25.2048)
  line L2669 (20.2612, 25.2048) -> (20.2612, 26.2048)
  line L2670 (20.2612, 26.2048) -> (19.2612, 26.2048)
  line L2671 (19.2612, 26.2048) -> (19.2612, 25.2048)
  line L2672 (19.8708, 25.2048) -> (20.8708, 25.2048)
  line L2673 (20.8708, 25.2048) -> (20.8708, 26.2048)
  line L2674 (20.8708, 26.2048) -> (19.8708, 26.2048)
  line L2675 (19.8708, 26.2048) -> (19.8708, 25.2048)
  line L2676 (20.4804, 25.2048) -> (21.4804, 25.2048)
  line L2677 (21.4804, 25.2048) -> (21.4804, 26.2048)
  line L2678 (21.4804, 26.2048) -> (20.4804, 26.2048)
  line L2679 (20.4804, 26.2048) -> (20.4804, 25.2048)
  line L2680 (21.2678, 25.2048) -> (22.2678, 25.2048)
  line L2681 (22.2678, 25.2048) -> (22.2678, 26.2048)
  line L2682 (22.2678, 26.2048) -> (21.2678, 26.2048)
  line L2683 (21.2678, 26.2048) -> (21.2678, 25.2048)
  line L2684 (21.725, 25.2048) -> (22.725, 25.2048)
  line L2685 (22.725, 25.2048) -> (22.725, 26.2048)
  line L2686 (22.725, 26.2048) -> (21.725, 26.2048)
  line L2687 (21.725, 26.2048) -> (21.725, 25.2048)
  line L2688 (12.8731, 25.2302) -> (13.8731, 25.2302)
  line L2689 (13.8731, 25.2302) -> (13.8731, 26.2302)
  line L2690 (13.8731, 26.2302) -> (12.8731, 26.2302)
  line L2691 (12.8731, 26.2302) -> (12.8731, 25.2302)
  line L2692 (13.9319, 25.7175) -> (13.9573, 25.7175)
  line L2693 (13.9573, 25.7175) -> (13.9573, 25.7429)
  line L2694 (13.9573, 25.7429) -> (13.9319, 25.7429)
  line L2695 (13.9319, 25.7429) -> (13.9319, 25.7175)
  line L2696 (14.5241, 25.2302) -> (15.5241, 25.2302)
  line L2697 (15.5241, 25.2302) -> (15.5241, 26.2302)
  line L2698 (15.5241, 26.2302) -> (14.5241, 26.2302)
  line L2699 (14.5241, 26.2302) -> (14.5241, 25.2302)
  line L2700 (15.4893, 25.2302) -> (16.4893, 25.2302)
  line L2701 (16.4893, 25.2302) -> (16.4893, 26.2302)
  line L2702 (16.4893, 26.2302) -> (15.4893, 26.2302)
  line L2703 (15.4893, 26.2302) -> (15.4893, 25.2302)
  line L2704 (16.2386, 25.2302) -> (17.2386, 25.2302)
  line L2705 (17.2386, 25.2302) -> (17.2386, 26.2302)
  line L2706 (17.2386, 26.2302) -> (16.2386, 26.2302)
  line L2707 (16.2386, 26.2302) -> (16.2386, 25.2302)
  line L2708 (17.0768, 25.2302) -> (18.0768, 25.2302)
  line L2709 (18.0768, 25.2302) -> (18.0768, 26.2302)
  line L2710 (18.0768, 26.2302) -> (17.0768, 26.2302)
  line L2711 (17.0768, 26.2302) -> (17.0768, 25.2302)
  line L2712 (17.9658, 25.2302) -> (18.9658, 25.2302)
  line L2713 (18.9658, 25.2302) -> (18.9658, 26.2302)
  line L2714 (18.9658, 26.2302) -> (17.9658, 26.2302)
  line L2715 (17.9658, 26.2302) -> (17.9658, 25.2302)
  line L2716 (18.6897, 25.2302) -> (19.6897, 25.2302)
  line L2717 (19.6897, 25.2302) -> (19.6897, 26.2302)
  line L2718 (19.6897, 26.2302) -> (18.6897, 26.2302)
  line L2719 (18.6897, 26.2302) -> (18.6897, 25.2302)
  line L2720 (19.2612, 25.2302) -> (20.2612, 25.2302)
  line L2721 (20.2612, 25.2302) -> (20.2612, 26.2302)
  line L2722 (20.2612, 26.2302) -> (19.2612, 26.2302)
  line L2723 (19.2612, 26.2302) -> (19.2612, 25.2302)
  line L2724 (19.8581, 25.2302) -> (20.8581, 25.2302)
  line L2725 (20.8581, 25.2302) -> (20.8581, 26.2302)
  line L2726 (20.8581, 26.2302) -> (19.8581, 26.2302)
  line L2727 (19.8581, 26.2302) -> (19.8581, 25.2302)
  line L2728 (20.4804, 25.2302) -> (21.4804, 25.2302)
  line L2729 (21.4804, 25.2302) -> (21.4804, 26.2302)
  line L2730 (21.4804, 26.2302) -> (20.4804, 26.2302)
  line L2731 (20.4804, 26.2302) -> (20.4804, 25.2302)
  line L2732 (21.2678, 25.2302) -> (22.2678, 25.2302)
  line L2733 (22.2678, 25.2302) -> (22.2678, 26.2302)
  line L2734 (22.2678, 26.2302) -> (21.2678, 26.2302)
  line L2735 (21.2678, 26.2302) -> (21.2678, 25.2302)
  line L2736 (21.7504, 25.2302) -> (22.7504, 25.2302)
  line L2737 (22.7504, 25.2302) -> (22.7504, 26.2302)
  line L2738 (22.7504, 26.2302) -> (21.7504, 26.2302)
  line L2739 (21.7504, 26.2302) -> (21.7504, 25.2302)
  line L2740 (12.8731, 25.2556) -> (13.8731, 25.2556)
  line L2741 (13.8731, 25.2556) -> (13.8731, 26.2556)
  line L2742 (13.8731, 26.2556) -> (12.8731, 26.2556)
  line L2743 (12.8731, 26.2556) -> (12.8731, 25.2556)
  line L2744 (14.5495, 25.2556) -> (15.5495, 25.2556)
  line L2745 (15.5495, 25.2556) -> (15.5495, 26.2556)
  line L2746 (15.5495, 26.2556) -> (14.5495, 26.2556)
  line L2747 (14.5495, 26.2556) -> (14.5495, 25.2556)
  line L2748 (15.4893, 25.2556) -> (16.4893, 25.2556)
  line L2749 (16.4893, 25.2556) -> (16.4893, 26.2556)
  line L2750 (16.4893, 26.2556) -> (15.4893, 26.2556)
  line L2751 (15.4893, 26.2556) -> (15.4893, 25.2556)
  line L2752 (16.2386, 25.2556) -> (17.2386, 25.2556)
  line L2753 (17.2386, 25.2556) -> (17.2386, 26.2556)
  line L2754 (17.2386, 26.2556) -> (16.2386, 26.2556)
  line L2755 (16.2386, 26.2556) -> (16.2386, 25.2556)
  line L2756 (17.0768, 25.2556) -> (18.0768, 25.2556)
  line L2757 (18.0768, 25.2556) -> (18.0768, 26.2556)
  line L2758 (18.0768, 26.2556) -> (17.0768, 26.2556)
  line L2759 (17.0768, 26.2556) -> (17.0768, 25.2556)
  line L2760 (17.9658, 25.2556) -> (18.9658, 25.2556)
  line L2761 (18.9658, 25.2556) -> (18.9658, 26.2556)
  line L2762 (18.9658, 26.2556) -> (17.9658, 26.2556)
  line L2763 (17.9658, 26.2556) -> (17.9658, 25.2556)